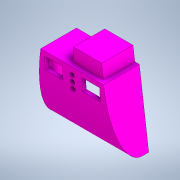
# Autodesk Inventor part: hull_electronics_top
Saved by Autodesk Inventor 2020 (Build 240168000, 168)
## iProperties
Created: 2019-09-19
Part Number: hull_electronics_top
Material: Generic
Document SubType Name: Modeling
Designer: suchanek
Density: 1 g/cm^3
Appearance: Default
Author: suchanek
Autodesk Inventor part; units mm, degrees
sketch "Sketch1" plane through (0, 0, 0) normal (0, 0, 1) x (1, 0, 0)
  line L0 (27.8975, 30) -> (32.9406, 30) projected
  line L1 (32.9406, 30) -> (42.8145, -45) projected
  line L2 (42.8145, -45) -> (-42.8145, -45) projected
  line L3 (-42.8145, -45) -> (-32.9406, 30) projected
  line L4 (-32.9406, 30) -> (-1, 30) projected
  line L5 (-1, 30) -> (-1, 45) projected
  line L6 (-1, 45) -> (25.9227, 45) projected
  line L7 (25.9227, 45) -> (27.8975, 30) projected
  line L8 (-45.6652, -47.5) -> (45.6652, -47.5) projected
  line L9 (45.6652, -47.5) -> (35.133, 32.5) projected
  line L10 (35.133, 32.5) -> (30.0899, 32.5) projected
  line L11 (30.0899, 32.5) -> (28.1151, 47.5) projected
  line L12 (28.1151, 47.5) -> (-3.5, 47.5) projected
  line L13 (-3.5, 47.5) -> (-3.5, 32.5) projected
  line L14 (-3.5, 32.5) -> (-35.133, 32.5) projected
  line L15 (-35.133, 32.5) -> (-45.6652, -47.5) projected
  point P0 (0, 0)
ref_plane "Work Plane1" through (-42.8145, -45, 6) normal (0, 0, 1) x (1, 0, 0)
extrude "Extrusion1" add sketch "Sketch1" along normal up to surface (6 mm away)
sketch "Sketch2" plane through (-45.6652, -47.5, 6) normal (0, 0, 1) x (1, 0, 0)
  line L0 (73.5627, 77.5) -> (71.5879, 92.5) projected
  line L1 (71.5879, 92.5) -> (44.6652, 92.5) projected
  line L2 (44.6652, 92.5) -> (44.6652, 77.5) projected
  line L3 (44.6652, 77.5) -> (12.7246, 77.5) projected
  line L4 (12.7246, 77.5) -> (2.8507, 2.5) projected
  line L5 (2.8507, 2.5) -> (88.4798, 2.5) projected
  line L6 (88.4798, 2.5) -> (78.6059, 77.5) projected
  line L7 (78.6059, 77.5) -> (73.5627, 77.5) projected
  line L8 (76.4134, 75) -> (85.6291, 5) projected
  line L9 (85.6291, 5) -> (5.7014, 5) projected
  line L10 (5.7014, 5) -> (14.9171, 75) projected
  line L11 (14.9171, 75) -> (47.1652, 75) projected
  line L12 (47.1652, 75) -> (47.1652, 90) projected
  line L13 (47.1652, 90) -> (69.3955, 90) projected
  line L14 (69.3955, 90) -> (71.3703, 75) projected
  line L15 (71.3703, 75) -> (76.4134, 75) projected
  line L16 (44.6652, 77.5) -> (12.7246, 77.5) projected
  line L17 (44.6652, 92.5) -> (44.6652, 77.5) projected
  line L18 (71.5879, 92.5) -> (44.6652, 92.5) projected
  line L19 (73.5627, 77.5) -> (71.5879, 92.5) projected
  line L20 (78.6059, 77.5) -> (73.5627, 77.5) projected
  line L21 (88.4798, 2.5) -> (78.6059, 77.5) projected
  line L22 (2.8507, 2.5) -> (88.4798, 2.5) projected
  line L23 (12.7246, 77.5) -> (2.8507, 2.5) projected
  line L24 (73.7804, 95) -> (75.7552, 80) projected
  line L25 (42.1652, 95) -> (73.7804, 95) projected
  line L26 (42.1652, 80) -> (42.1652, 95) projected
  line L27 (10.5322, 80) -> (42.1652, 80) projected
  line L28 (0, 0) -> (10.5322, 80) projected
  line L29 (91.3305, 0) -> (0, 0) projected
  line L30 (80.7983, 80) -> (91.3305, 0) projected
  line L31 (75.7552, 80) -> (80.7983, 80) projected
  point P0 (45.6652, 47.5)
extrude "Extrusion2" add sketch "Sketch2" along normal blind 1 contours L7 L6 L5 L4 L3 L2 L1 L0 | L24 L31 L30 L29 L28 L27 L26 L25
sketch "Sketch3" plane through (-45.6652, -47.5, 7) normal (0, 0, 1) x (1, 0, 0)
  line L0 (75.7552, 80) -> (73.7804, 95) projected
  line L1 (73.7804, 95) -> (42.1652, 95) projected
  line L2 (42.1652, 95) -> (42.1652, 80) projected
  line L3 (42.1652, 80) -> (10.5322, 80) projected
  line L4 (10.5322, 80) -> (0, 0) projected
  line L5 (0, 0) -> (91.3305, 0) projected
  line L6 (91.3305, 0) -> (80.7983, 80) projected
  line L7 (80.7983, 80) -> (75.7552, 80) projected
  line L8 (71.3703, 75) -> (76.4134, 75) projected
  line L9 (76.4134, 75) -> (85.6291, 5) projected
  line L10 (85.6291, 5) -> (5.7014, 5) projected
  line L11 (5.7014, 5) -> (14.9171, 75) projected
  line L12 (14.9171, 75) -> (47.1652, 75) projected
  line L13 (47.1652, 75) -> (47.1652, 90) projected
  line L14 (47.1652, 90) -> (69.3955, 90) projected
  line L15 (69.3955, 90) -> (71.3703, 75) projected
  line L16 (5.7014, 5) -> (14.9171, 75) projected
  line L17 (5.7014, 5) -> (5.0431, 0)
  line L18 (0, 0) -> (91.3305, 0) projected
  line L19 (85.6291, 5) -> (86.2874, 0)
  line L20 (5.0431, 0) -> (0, 0)
  line L21 (86.2874, 0) -> (91.3305, 0)
  point P0 (45.6652, 47.5)
  point P1 (5.0431, 0)
  constraints: 8 end point, 4 collinear, 2 point on line
ref_plane "Work Plane2" through (-35.133, 32.5, 40) normal (0, 0, 1) x (1, 0, 0)
extrude "Extrusion3" add sketch "Sketch3" along normal up to surface (33 mm away) contours L7 L6 L5 L19 L9 L8 L15 L14 L13 L12 L11 L17 L4 L3 L2 L1 L0
ref_plane "Work Plane3" through (-73.5, 32.5, 0) normal (-1, 0, 0) x (0, 0, 1)
sketch "Sketch4" plane through (-73.5, 32.5, 0) normal (-1, 0, 0) x (0, 0, 1)
  line L0 (-80, -60) -> (-85, -60) projected
  line L1 (-85, -60) -> (-85, -20) projected
  line L2 (-85, -20) -> (-80, -20) projected
  line L3 (-80, 0) -> (-80, -20) projected
  line L4 (-80, 0) -> (40, 0) projected
  line L5 (40, 20) -> (40, 0) projected
  line L6 (-95, 20) -> (40, 20) projected
  line L7 (-95, -80) -> (-95, 20) projected
  line L8 (-80, -80) -> (-95, -80) projected
  line L9 (-80, -60) -> (-80, -80) projected
  line L10 (0, 0) -> (40, 0) projected
  line L11 (0, 0) -> (0, -80) projected
  line L12 (0, -80) -> (40, -80) projected
  line L13 (40, -80) -> (40, 0) projected
  line L14 (35, 15) -> (35, 0) projected
  line L15 (0, 0) -> (40, 0) projected
  line L16 (35, 15) -> (40, 15)
  line L17 (40, 15) -> (40, 0)
  line L18 (40, 0) -> (35, 0)
  line L19 (35, 0) -> (35, 15)
  line L20 (0, 0) -> (0, -80) projected
  line L21 (40, -80) -> (40, 0) projected
  line L22 (7, -75) -> (7, -80) projected
  line L23 (7, -80) -> (40, -80)
  line L24 (7, -80) -> (7, 0)
  ellipse E0 centre (7, 0) end of major axis (7, -80) minor radius 33
  line L25 (0, -80) -> (40, -80) projected
  point P0 (0, -32.5)
  point P1 (40, 0)
  point P2 (40, 0)
  constraints: 12 end point, 3 horizontal, 2 parallel, 2 perpendicular, 1 coincident, 1 point on line, 4 other
extrude "Extrusion4" cut sketch "Sketch4" against normal through all contours E0 L4 L14 L16 | L16 L5 E0 | E0 L13 L12
sketch "Sketch7" plane through (-3.5, 32.5, 0) normal (-1, 0, 0) x (0, 0, 1)
  line L0 (35, 0) -> (35, 15) projected
  line L1 (0, 0) -> (40, 0) projected
  line L2 (35, 15) -> (30, 15)
  line L3 (30, 15) -> (30, 0)
  line L4 (30, 0) -> (35, 0)
  line L5 (35, 0) -> (35, 15)
  line L6 (30, 0) -> (35, 0)
  line L7 (35, 0) -> (35, -5)
  line L8 (35, -5) -> (30, -5)
  line L9 (30, -5) -> (30, 0)
  point P0 (0, -32.5)
  dimension "d9" = 5
  dimension "d10" = 5
  constraints: 16 end point, 4 parallel, 2 horizontal, 2 perpendicular, 1 collinear, 1 point on line
  measures "d9" distance of L4.end L3.end
  measures "d10" distance of L6.end L7.end
extrude "Extrusion5" add sketch "Sketch7" against normal up to surface (31.6151 mm away)
sketch "Sketch14" plane through (-73.5, 32.5, 0) normal (-1, 0, 0) x (0, 0, 1)
  ellipse E0 centre (7, 0) end of major axis (7, 80) minor radius 33 (7, -80) -> (40, 0) ccw projected
  line L0 (40, 0) -> (36, 0)
  line L1 (7, -76) -> (7, -80)
  line L2 (0, -2.5) -> (0, -77.5) projected
  spline S0 degree 5 poles (7, -76.0001) (7.0916, -76.0001) (7.1831, -75.999) (7.2747, -75.9968) (8.7132, -75.9454) (10.1393, -75.6245) (11.4029, -75.1078) (14.3005, -73.5105) (16.7621, -71.2736) (18.0817, -69.8362) (20.9474, -66.2285) (23.2953, -62.2605) (24.5174, -59.9036) (26.9909, -54.5266) (28.977, -48.9488) (29.9505, -45.8318) (31.7991, -39.1047) (33.199, -32.2694) (33.8313, -28.6116) (34.9214, -21.0246) (35.5888, -13.3884) (35.8269, -9.4416) (35.9723, -5.1828) (35.9981, -0.923) (35.9994, -0.6153) (36, -0.3077) (36, 0) knots 0 0 0 0 0 0 0.005302 0.005302 0.005302 0.083325 0.083325 0.083325 0.196068 0.196068 0.196068 0.349565 0.349565 0.349565 0.538506 0.538506 0.538506 0.753333 0.753333 0.753333 0.982185 0.982185 0.982185 1 1 1 1 1 1
  point P0 (0, -32.5)
  dimension "d16" = 4
  constraints: 4 end point, 1 horizontal, 1 parallel, 5 other
extrude "Extrusion6" add sketch "Sketch14" against normal through all
sketch "Sketch15" plane through (0, 0, 0) normal (0, 0, -1) x (-1, 0, 0)
  line L0 (-28.1151, 47.5) -> (3.5, 47.5) projected
  line L1 (-30.0899, 32.5) -> (-28.1151, 47.5) projected
  line L2 (-35.133, 32.5) -> (-30.0899, 32.5) projected
  line L3 (-45.6652, -47.5) -> (-35.133, 32.5) projected
  line L4 (45.6652, -47.5) -> (-45.6652, -47.5) projected
  line L5 (35.133, 32.5) -> (45.6652, -47.5) projected
  line L6 (3.5, 32.5) -> (35.133, 32.5) projected
  line L7 (3.5, 47.5) -> (3.5, 32.5) projected
  line L8 (1, 30) -> (1, 45) projected
  line L9 (32.9406, 30) -> (1, 30) projected
  line L10 (42.8145, -45) -> (32.9406, 30) projected
  line L11 (-42.8145, -45) -> (42.8145, -45) projected
  line L12 (-32.9406, 30) -> (-42.8145, -45) projected
  line L13 (-27.8975, 30) -> (-32.9406, 30) projected
  line L14 (-25.9227, 45) -> (-27.8975, 30) projected
  line L15 (1, 45) -> (-25.9227, 45) projected
  point P0 (0, 0)
extrude "Extrusion7" cut sketch "Sketch15" against normal through all contours L0 L7 L6 L5 L4 L3 L2 L1 | L9 L10 L11 L12 L13 L14 L15 L8 keep common part
ref_plane "Work Plane4" through (35.133, 32.5, 40) normal (0, 0, 1) x (1, 0, 0)
sketch "Sketch16" plane through (35.133, 32.5, 40) normal (0, 0, 1) x (1, 0, 0)
  line L0 (-4.3849, -5) -> (-24.1849, -5)
  line L1 (-24.1849, -5) -> (-24.1849, -18.8)
  line L2 (-24.1849, -18.8) -> (-4.3849, -18.8)
  line L3 (-4.3849, -18.8) -> (-4.3849, -5)
  line L4 (-75.0969, -75) -> (-65.8812, -5) projected
  line L5 (-65.8812, -5) -> (-46.0812, -5)
  line L6 (-46.0812, -5) -> (-46.0812, -18.8)
  line L7 (-46.0812, -18.8) -> (-65.8812, -18.8)
  line L8 (-65.8812, -18.8) -> (-65.8812, -5)
  circle A0 centre (-35.133, -8) radius 2.5
  line L9 (-35.133, -8) -> (-35.133, -7.9793)
  circle A1 centre (-35.133, -15) radius 2.5
  circle A2 centre (-35.133, -22) radius 2.5
  point P0 (-35.133, -32.5)
  dimension "d21" = 19.8
  dimension "d22" = 13.8
  dimension "d23" = 19.8
  dimension "d24" = 13.8
  dimension "d25" = 5
  dimension "d29" = 7
  dimension "d34" = 3
  constraints: 18 end point, 4 parallel, 3 centre point, 2 horizontal, 2 perpendicular, 1 coincident, 1 vertical, 5 other
  measures "d21" distance of L2.end L1.end
  measures "d22" distance of L1.end L0.end
  measures "d23" distance of L6.end L7.end
  measures "d24" distance of L5.end L6.end
  measures "d25" diameter of A0
  measures "d29" distance of L9.start A1.centre
  measures "d34" distance from line of L0 L9.start
extrude "Extrusion8" cut sketch "Sketch16" against normal blind 10
sketch "Sketch17" plane through (-3.5, 47.5, 35) normal (0, 0, 1) x (1, 0, 0)
  line L0 (0, -15) -> (0, 0) projected
  line L1 (0, -15) -> (34.2482, -15)
  line L2 (34.2482, -15) -> (34.2482, -20)
  line L3 (34.2482, -20) -> (0, -20)
  line L4 (0, -20) -> (0, -15)
  point P0 (3.5, -47.5)
  constraints: 8 end point, 2 parallel, 1 horizontal, 1 perpendicular
extrude "Extrusion9" add sketch "Sketch17" along normal blind 3
equation "\"d23\" = d21"
equation "\"d24\" = d22"
body "Solid1"
